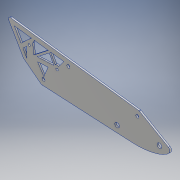
# Autodesk Inventor part: bracket1
Saved by Autodesk Inventor 2018.2 (Build 222227000, 227)
## iProperties
Created: 2018-03-05
Part Number: bracket1
Material: アルミニウム 6061
Document SubType Name: Modeling
Designer: ku_sk
Density: 2.7 g/cm^3
Appearance: アルミニウム - フラット
Mass: 349.891 g
Surface Area: 692.084 cm^2
Volume: 129.589 cm^3
Author: ku_sk
Autodesk Inventor part; units mm, degrees
ref_plane "YZ Plane" through (0, 0, 0) normal (1, 0, 0) x (0, 1, 0)
ref_plane "XZ Plane" through (0, 0, 0) normal (0, 1, 0) x (-1, 0, 0)
ref_plane "XY Plane" through (0, 0, 0) normal (0, 0, 1) x (1, 0, 0)
sketch "スケッチ2" plane through (0, 0, 0) normal (0, 1, 0) x (-1, 0, 0)
  arc A0 (320.7468, 34.8983) -> (392.1215, 71.6787) centre (243.1623, 273.099) ccw projected
  arc A1 (310.5095, 31.8959) -> (320.7468, 34.8983) centre (264.9264, 206.2785) ccw projected
  arc A2 (290.9118, 29.5172) -> (310.5095, 31.8959) centre (291.9468, 102.9093) ccw projected
  arc A3 (278.6891, 31.4878) -> (290.9118, 29.5172) centre (291.5128, 72.1352) ccw projected
  arc A4 (274.9831, 33.389) -> (278.6891, 31.4878) centre (282.4278, 43.3382) ccw projected
  arc A5 (275.4733, 39.2078) -> (274.9831, 33.389) centre (277.0456, 36.1453) ccw projected
  arc A6 (283.1253, 42.3274) -> (275.4733, 39.2078) centre (297.1464, -3.0086) ccw projected
  arc A7 (310.1184, 49.282) -> (283.1253, 42.3274) centre (369.3413, -236.446) ccw projected
  arc A8 (310.1184, 49.282) -> (326.9533, 52.7997) centre (-771.7798, 5269.0252) ccw projected
  arc A9 (326.9533, 52.7997) -> (357.98, 60.8795) centre (256.8539, 385.5961) ccw projected
  arc A10 (357.98, 60.8795) -> (391.1188, 73.3957) centre (268.9975, 346.6028) ccw projected
  arc A11 (392.1215, 71.6787) -> (391.1188, 73.3957) centre (391.5269, 72.4828) ccw projected
  circle A12 centre (287.1934, 37.1564) radius 3 projected
  circle A13 centre (359.7933, 56.2153) radius 3 projected
  arc A14 (100.5026, -29.4375) -> (303.8176, 17.6729) centre (68.6386, 570.3585) ccw projected
  arc A15 (74.9408, -30.0377) -> (100.5026, -29.4375) centre (77.5861, 401.9345) ccw projected
  arc A16 (28.1912, -23.4013) -> (74.9408, -30.0377) centre (76.0159, 145.5175) ccw projected
  arc A17 (1.2395, -11.312) -> (28.1912, -23.4013) centre (55.8939, 74.446) ccw projected
  arc A18 (-6.0217, -4.7376) -> (1.2395, -11.312) centre (16.9451, 13.3315) ccw projected
  arc A19 (-1.6159, 7.4897) -> (-6.0217, -4.7376) centre (0, 0) ccw projected
  arc A20 (17.9572, 9.9554) -> (-1.6159, 7.4897) centre (22.277, -103.2534) ccw projected
  arc A21 (84.7958, 9.311) -> (17.9572, 9.9554) centre (44.6377, -689.2581) ccw projected
  arc A22 (84.7958, 9.311) -> (126.0099, 7.0084) centre (819.0754, 12782.4716) ccw projected
  arc A23 (126.0099, 7.0084) -> (203.0122, 6.466) centre (170.258, 822.6468) ccw projected
  arc A24 (203.0122, 6.466) -> (303.8176, 17.6729) centre (174.1884, 724.7085) ccw projected
  circle A25 centre (20.0666, -1.5588) radius 5 projected
  circle A26 centre (130.4331, -10.1322) radius 5 projected
  line L0 (100.5026, -29.4375) -> (327.9026, -17.3569)
  line L1 (-3.831, 6.6355) -> (72.6844, 50.8117)
  line L2 (1137.2465, 0) -> (-1089.9509, 0) projected
  line L3 (72.6844, 50.8117) -> (483.7253, 102.9093)
  line L4 (327.9026, -17.3569) -> (483.7253, 102.9093)
  point P0 (0, 0)
  point P1 (371.2778, 57.8193)
  dimension "d7" = 30
  constraints: 8 end point, 2 point on circle, 2 tangent
  measures "d7" angle of L2 L1
extrude "押し出し3" add sketch "スケッチ2" along normal blind 4 contours A1 A2 A3 A4 A5 A6 A7 A8 A9 A10 A11 A0 | A15 A16 A17 A18 A19 L2 A25 A14 | A14 L2 L4 L0 | L2 A25 A19 A20 A21 A22 A23 A24 A14 | A14 A24 A23 A22 A21 A20 A19 L1 L3 L4 L2
sketch "スケッチ3" plane through (0, 4, 0) normal (0, 1, 0) x (1, 0, 0)
  line L0 (-483.7253, -102.9093) -> (-72.6844, -50.8117) projected
  line L1 (-327.9026, 17.3569) -> (-483.7253, -102.9093) projected
  line L2 (-483.7253, -102.9093) -> (-72.6844, -50.8117) projected
  line L3 (-418.3387, -94.6218) -> (-374.803, -18.8415)
  line L4 (-327.9026, 17.3569) -> (-483.7253, -102.9093) projected
  point P0 (0, 0)
  constraints: 2 end point, 2 point on line
extrude "押し出し4" cut sketch "スケッチ3" against normal through all
fillet "フィレット2" radius 5 4 edges at (-418.3387, 2, 94.6218) (-72.6844, 2, 50.8117) (-327.9026, 2, -17.3569) (-374.803, 2, 18.8415)
sketch "スケッチ4" plane through (0, 4, 0) normal (0, 1, 0) x (1, 0, 0)
  circle A0 centre (-77.5679, -36.3106) radius 4
  circle A1 centre (-322.4385, 2.626) radius 4
  circle A2 centre (-257.5679, -59.1248) radius 4
  line L0 (-71.8122, -50.3081) -> (3.831, -6.6355) projected
  line L1 (-408.3679, -93.358) -> (-73.6835, -50.9383) projected
  line L2 (-100.5026, 29.4375) -> (-326.3465, 17.4396) projected
  line L3 (-329.1362, 16.4048) -> (-374.0171, -18.2349) projected
  point P0 (0, 0)
  dimension "d15" = 15
  dimension "d16" = 15
  dimension "d17" = 8
  dimension "d18" = 15
  dimension "d19" = 8
  dimension "d20" = 180
  dimension "d21" = 8
  dimension "d22" = 15
  dimension "d23" = 15
  constraints: 3 centre point
  measures "d15" distance from line of L0 A0.centre
  measures "d16" distance from line of A0.centre L1
  measures "d17" diameter of A0
  measures "d18" distance from line of L1 A2.centre
  measures "d19" diameter of A2
  measures "d20" horizontal distance of A0.centre A2.centre
  measures "d21" diameter of A1
  measures "d22" distance from line of L2 A1.centre
  measures "d23" distance from line of L3 A1.centre
extrude "押し出し5" cut sketch "スケッチ4" against normal through all
sketch "スケッチ5" plane through (0, 0, 0) normal (0, -1, 0) x (1, 0, 0)
  line L0 (-398.4053, 79.9993) -> (-354.2225, 74.3994)
  line L1 (-354.2225, 74.3994) -> (-380.9703, 49.651)
  line L2 (-380.9703, 49.651) -> (-398.4053, 79.9993)
  line L3 (-408.3679, 93.358) -> (-73.6835, 50.9383) projected
  line L4 (-413.332, 85.907) -> (-375.2976, 19.7024) projected
  line L5 (-365.897, 23.4137) -> (-375.8599, 40.7556)
  line L6 (-375.8599, 40.7556) -> (-365.84, 50.0265)
  line L7 (-365.84, 50.0265) -> (-365.897, 23.4137)
  line L8 (-309.8713, 68.7781) -> (-346.1762, 73.3795)
  line L9 (-309.8713, 68.7781) -> (-347.3681, 39.7172)
  line L10 (-347.3681, 39.7172) -> (-350.7508, 64.4872)
  line L11 (-338.6611, 40.1394) -> (-307.5903, 64.22)
  line L12 (-307.5903, 64.22) -> (-295.7115, 42.2224)
  line L13 (-295.7115, 42.2224) -> (-338.6611, 40.1394)
  line L14 (-303.9651, 68.0295) -> (-269.4979, 63.6609)
  line L15 (-269.4979, 63.6609) -> (-282.8063, 46.1427)
  arc A0 (-282.8063, 46.1427) -> (-292.0222, 45.9133) centre (-287.1934, 37.1564) ccw
  line L16 (-303.9651, 68.0295) -> (-292.0222, 45.9133)
  circle A1 centre (-287.1934, 37.1564) radius 3 projected
  line L17 (-346.1762, 73.3795) -> (-350.7508, 64.4872)
  line L18 (-337.7036, 29.1729) -> (-310.6204, 30.4864)
  line L19 (-310.6204, 30.4864) -> (-321.4627, 3.9493)
  line L20 (-321.4627, 3.9493) -> (-337.7036, 29.1729)
  point P0 (0, 0)
  dimension "d35" = 12
  dimension "d36" = 10
  dimension "d39" = 10
  dimension "d40" = 35
  dimension "d41" = 50
  dimension "d42" = 30
  dimension "d43" = 20
  dimension "d46" = 5
  dimension "d56" = 35
  dimension "d57" = 5
  dimension "d58" = 7
  dimension "d59" = 25
  dimension "d60" = 43
  dimension "d61" = 60
  dimension "d62" = 22
  dimension "d63" = 110
  dimension "d64" = 8.1107
  dimension "d65" = 60
  dimension "d66" = 10
  dimension "d67" = 25
  dimension "d68" = 145
  dimension "d69" = 11
  dimension "d70" = 60
  dimension "d71" = 65
  dimension "d72" = 30
  constraints: 38 end point, 7 parallel, 3 collinear, 2 point on circle, 1 centre point, 1 concentric, 1 point on line
  measures "d35" distance between parallel lines of L0 L3
  measures "d36" distance between parallel lines of L4 L2
  measures "d39" distance between parallel lines of L1 L6
  measures "d40" distance of L1.end L0.start
  measures "d41" angle of L1 L0
  measures "d42" angle of L5 L7
  measures "d43" distance of L5.start L5.end
  measures "d46" distance between parallel lines of L11 L9
  measures "d56" angle of L13 L11
  measures "d57" distance between parallel lines of L12 L16
  measures "d58" radial gap between concentric circles of A1 A0
  measures "d59" distance of L11.end L12.end
  measures "d60" distance of L12.end L11.start
  measures "d61" angle of L15 L14
  measures "d62" distance of L14.end L15.end
  measures "d63" angle of L8 L17
  measures "d64" distance of L0.end L8.end
  measures "d65" angle of L9 L10
  measures "d66" distance of L8.end L10.end
  measures "d67" distance of L9.end L10.end
  measures "d68" angle of L10 L17
  measures "d69" distance between parallel lines of L18 L13
  measures "d70" angle of L20 L18
  measures "d71" angle of L19 L18
  measures "d72" distance of L19.end L18.start
sketch "スケッチ6" plane through (0, 0, 0) normal (0, -1, 0) x (1, 0, 0)
  circle A0 centre (-20.0666, -1.5588) radius 6
  circle A1 centre (-20.0666, -1.5588) radius 5 projected
  circle A2 centre (-130.4331, -10.1322) radius 6
  circle A3 centre (-130.4331, -10.1322) radius 5 projected
  point P0 (0, 0)
  dimension "d29" = 12
  dimension "d30" = 12
  constraints: 2 centre point, 2 concentric
  measures "d29" diameter of A0
  measures "d30" diameter of A2
extrude "押し出し7" cut sketch "スケッチ6" against normal through all
extrude "押し出し8" cut sketch "スケッチ5" against normal through all contours L0 L1 L2 | L5 L6 L7 | L9 L10 L17 L8 | L11 L12 L13 | L14 L15 A0 L16 | L18 L19 L20
equation "\"d16\" = d15"
equation "\"d18\" = d16"
equation "\"d19\" = d17"
equation "\"d21\" = d19"
equation "\"d22\" = d18"
equation "\"d23\" = d22"
